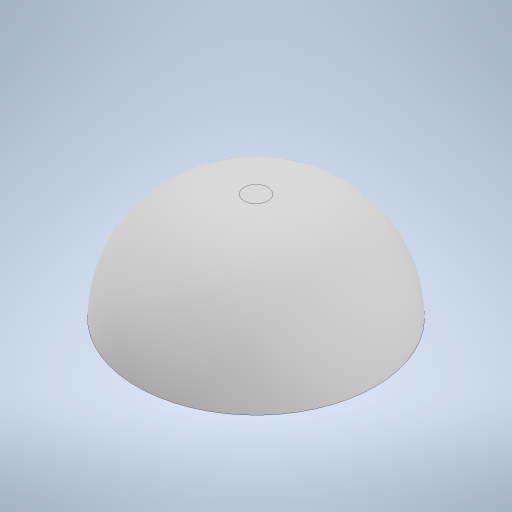
# Autodesk Inventor part: Kulka
Saved by Autodesk Inventor 2023 (Build 270158000, 158)
## iProperties
Created: 2023-02-09
Part Number: Kulka
Material: Ogólny
Document SubType Name: Modeling
Designer: User
Density: 1 g/cm^3
Appearance: Domyślna
Author: User
Autodesk Inventor part; units mm, degrees
ref_plane "YZ Plane" through (0, 0, 0) normal (1, 0, 0) x (0, 1, 0)
ref_plane "XZ Plane" through (0, 0, 0) normal (0, 1, 0) x (-1, 0, 0)
ref_plane "XY Plane" through (0, 0, 0) normal (0, 0, 1) x (1, 0, 0)
sketch "Szkic2" plane through (0, 0, 0) normal (0, 1, 0) x (-1, 0, 0)
  line L0 (0, 0) -> (-10, 0)
  line L1 (-10, 0) -> (-10, -10)
  line L2 (-10, -10) -> (0, -10)
  line L3 (0, -10) -> (0, 0)
  circle A0 centre (-5, -5) radius 5
  dimension "d14" = 10
  dimension "d15" = 10
  constraints: 8 end point, 2 parallel, 2 tangent, 1 centre point, 1 horizontal, 1 perpendicular
  measures "d14" distance of L2.end L0.start
  measures "d15" distance of L1.end L2.end
sketch "Szkic2 outline for Wyciągnięcie proste4" plane through (0, 0, 0) normal (0, 1, 0) x (-1, 0, 0)
  circle A0 centre (-5, -5) radius 5
extrude "Wyciągnięcie proste4" add sketch "Szkic2 outline for Wyciągnięcie proste4" along normal blind 4.5
fillet "Zaokrąglenie1" radius 4.5 1 edges at (10, 4.5, -5)
